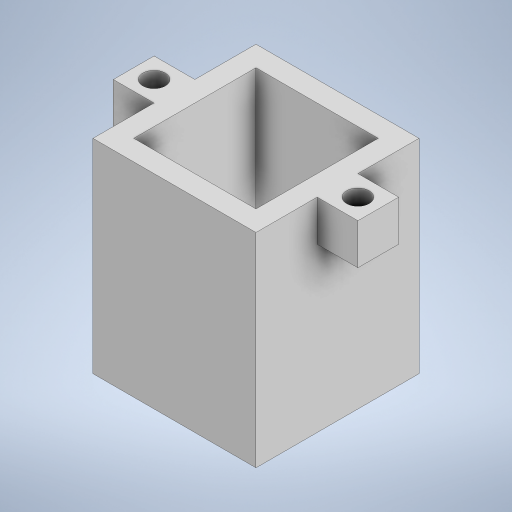
# Autodesk Inventor part: battery5V_box
Saved by Autodesk Inventor 2023 (Build 270158000, 158)
## iProperties
Created: 2023-05-22
Part Number: battery5V_box
Material: 一般
Document SubType Name: Modeling
Designer: 310611102
Density: 1 g/cm^3
Appearance: 預設
Author: 310611102
Autodesk Inventor part; units mm, degrees
ref_plane "YZ Plane" through (0, 0, 0) normal (1, 0, 0) x (0, 1, 0)
ref_plane "XZ Plane" through (0, 0, 0) normal (0, 1, 0) x (-1, 0, 0)
ref_plane "XY Plane" through (0, 0, 0) normal (0, 0, 1) x (1, 0, 0)
sketch "Sketch1" plane through (0, 0, 0) normal (0, 0, 1) x (1, 0, 0)
  line L0 (0, 0) -> (-40, 0)
  line L1 (-40, 0) -> (-40, 50)
  line L2 (-40, 50) -> (0, 50)
  line L3 (0, 50) -> (0, 0)
  dimension "d0" = 50
  dimension "d1" = 40
  constraints: 8 end point, 2 parallel, 1 horizontal, 1 perpendicular
  measures "d0" distance of L2.end L0.start
  measures "d1" distance of L1.end L2.end
extrude "Extrusion1" add sketch "Sketch1" along normal blind 40
sketch "Sketch2" plane through (-40, 50, 0) normal (0, 1, 0) x (1, 0, 0)
  line L0 (40, 0) -> (0, 0) projected
  line L1 (0, 0) -> (0, -40) projected
  line L2 (40, -40) -> (0, -40) projected
  line L3 (40, 0) -> (40, -40) projected
  line L4 (5, -5) -> (35, -5)
  line L5 (35, -5) -> (35, -35)
  line L6 (35, -35) -> (5, -35)
  line L7 (5, -35) -> (5, -5)
  dimension "d5" = 5
  constraints: 8 end point, 3 other
  measures "d5" distance between parallel lines of L0 L4
extrude "Extrusion2" cut sketch "Sketch2" against normal blind 30 contours L4 L5 L6 L7
sketch "Sketch3" plane through (-40, 0, 0) normal (0, -1, 0) x (1, 0, 0)
  circle A0 centre (5, 35) radius 2.5
  line L0 (5, 35) -> (7.3437, 35)
  line L1 (7.3437, 35) -> (7.3437, 32.7108)
  circle A1 centre (35, 35) radius 2.5
  circle A2 centre (5, 5) radius 2.5
  circle A3 centre (35, 5) radius 2.5
  line L2 (0, 40) -> (40, 40) projected
  line L3 (0, 0) -> (0, 40) projected
  point P0 (40, 0)
  dimension "d10" = 30
  dimension "d13" = 30
  dimension "d16" = 5
  dimension "d17" = 5
  dimension "d18" = 5
  constraints: 4 centre point, 4 end point, 2 horizontal, 1 perpendicular, 1 vertical, 6 other
  measures "d10" distance of L0.start A1.centre
  measures "d13" distance of L0.start A2.centre
  measures "d16" diameter of A0
  measures "d17" distance from line of L2 L0.start
  measures "d18" distance from line of L3 L0.start
extrude "Extrusion3" cut sketch "Sketch3" against normal blind 10
sketch "Sketch4" plane through (-40, 50, 0) normal (0, 1, 0) x (1, 0, 0)
  line L0 (0, 0) -> (0, -40) projected
  line L1 (0, -25) -> (-10, -25)
  line L2 (-10, -25) -> (-10, -15)
  line L3 (-10, -15) -> (0, -15)
  line L4 (0, -15) -> (0, -25)
  line L5 (40, 0) -> (40, -40) projected
  line L6 (40, -25) -> (50, -25)
  line L7 (50, -25) -> (50, -15)
  line L8 (50, -15) -> (40, -15)
  line L9 (40, -15) -> (40, -25)
  line L10 (-23.587, -20) -> (57.8749, -20)
  line L11 (40, -40) -> (0, -40) projected
  line L12 (35, -5) -> (35, -35) projected
  line L13 (35, -35) -> (5, -35) projected
  line L14 (5, -35) -> (5, -5) projected
  line L15 (5, -5) -> (35, -5) projected
  line L16 (40, 0) -> (0, 0) projected
  line L17 (0, 0) -> (0, -40) projected
  line L18 (40, -40) -> (0, -40) projected
  line L19 (40, 0) -> (40, -40) projected
  circle A0 centre (-5, -20) radius 2.75
  circle A1 centre (45, -20) radius 2.75
  point P0 (0, -20)
  point P1 (0, -20)
  point P2 (-5, -15)
  point P3 (45, -15)
  dimension "d21" = 10
  dimension "d22" = 10
  dimension "d23" = 10
  dimension "d26" = 5.5
  dimension "d27" = 5.5
  constraints: 18 end point, 7 point on line, 4 midpoint, 4 parallel, 3 horizontal, 2 centre point, 2 perpendicular, 2 vertical alignment, 2 other
  measures "d21" distance of L1.end L2.end
  measures "d22" distance of L2.end L3.end
  measures "d23" distance of L7.end L8.end
  measures "d26" diameter of A0
  measures "d27" diameter of A1
extrude "Extrusion4" add sketch "Sketch4" against normal blind 10 contours L0 L10 A0 L2 L3 | L0 L1 L2 L10 A0 | L8 L7 L10 A1 L5 | L10 A1 L7 L6 L5
body "Solid1"
